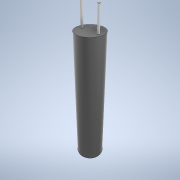
# Autodesk Inventor part: tds-sensor
Saved by Autodesk Inventor 2020.2 (Build 242310000, 310)
## iProperties
Created: 2020-05-08
Part Number: tds-sensor
Material: Generic
Document SubType Name: Modeling
Designer: Nicholas
Density: 1 g/cm^3
Appearance: Default
Author: Nicholas
Autodesk Inventor part; units mm, degrees
ref_plane "YZ Plane" through (0, 0, 0) normal (1, 0, 0) x (0, 1, 0)
ref_plane "XZ Plane" through (0, 0, 0) normal (0, 1, 0) x (-1, 0, 0)
ref_plane "XY Plane" through (0, 0, 0) normal (0, 0, 1) x (1, 0, 0)
sketch "Sketch1" plane through (0, 0, 0) normal (0, 1, 0) x (-1, 0, 0)
  circle A0 centre (0, 0) radius 3
  dimension "d0" = 6
  constraints: 1 centre point, 1 coincident
  measures "d0" diameter of A0
extrude "Extrusion1" add sketch "Sketch1" along normal blind 30
sketch "Sketch2" plane through (0, 30, 0) normal (0, 1, 0) x (1, 0, 0)
  circle A0 centre (0, 0) radius 3 construction
  line L0 (0, 3) -> (0, -3) construction
  line L1 (-3, 0) -> (3, 0) construction
  circle A1 centre (-2, 0) radius 0.25
  circle A2 centre (2, 0) radius 0.25
  dimension "d4" = 0.5
  dimension "d" = 2
  dimension "d6" = 4
  constraints: 4 end point, 4 point on circle, 2 centre point, 2 midpoint, 1 perpendicular, 1 point on line, 1 symmetric about line, 1 vertical, 1 other
  measures "d4" diameter of A1
  measures "d" distance from line of L0 A1.centre
  measures "d6" distance of A2.centre A1.centre
extrude "Extrusion2" add sketch "Sketch2" along normal blind 5
body "Solid1"
